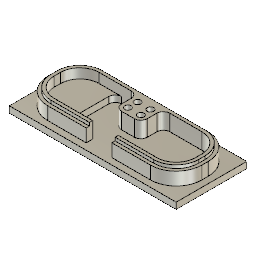
COURSERA01 (Autodesk Fusion 360 design; units mm, degrees)
Autodesk Fusion 360 part; units mm, degrees
sketch "Sketch1" plane through (0, 0, 0) normal (0, 0, 1) x (1, 0, 0)
  line L0 (-82.55, 34.925) -> (82.55, 34.925)
  line L1 (82.55, 34.925) -> (82.55, -34.925)
  line L2 (82.55, -34.925) -> (-82.55, -34.925)
  line L3 (-82.55, -34.925) -> (-82.55, 34.925)
  line L4 (-82.55, 34.925) -> (82.55, -34.925) construction
  line L5 (82.55, 34.925) -> (-82.55, -34.925) construction
  dimension "d1" = 165.1
  dimension "d2" = 69.85
  constraint horizontal L0
  constraint perpendicular L0 L1
  constraint parallel L0 L2
  constraint parallel L1 L3
  constraint coincident L4 origin
  constraint coincident L5 origin
  measures "d1" distance of L1.end L2.end
  measures "d2" distance of L0.end L1.end
extrude "Extrude1" add sketch "Sketch1" along normal blind 6.35
sketch "Sketch2" plane through (0, 0, 6.35) normal (0, 0, 1) x (-1, 0, 0)
  line L0 (82.55, 34.925) -> (-82.55, 34.925)
  line L1 (-82.55, 34.925) -> (-82.55, -34.925)
  line L2 (-82.55, -34.925) -> (82.55, -34.925)
  line L3 (82.55, -34.925) -> (82.55, 34.925)
sketch "Sketch3" plane through (0, 0, 6.35) normal (0, 0, 1) x (-1, 0, 0)
  line L0 (76.2, 28.575) -> (-76.2, 28.575)
  line L1 (-76.2, 28.575) -> (-76.2, -28.575)
  line L2 (-76.2, -28.575) -> (76.2, -28.575)
  line L3 (76.2, -28.575) -> (76.2, 28.575)
  line L4 (76.2, 28.575) -> (-76.2, -28.575) construction
  line L5 (-76.2, 28.575) -> (76.2, -28.575) construction
  dimension "d5" = 152.4
  dimension "d6" = 57.15
  constraint horizontal L0
  constraint perpendicular L0 L1
  constraint parallel L0 L2
  constraint parallel L1 L3
  constraint coincident L4 origin
  constraint coincident L5 origin
  measures "d5" distance of L1.end L2.end
  measures "d6" distance of L0.start L2.end
extrude "Extrude2" add sketch "Sketch3" along normal blind 12.7
sketch "Sketch4" plane through (0, 0, 19.05) normal (0, 0, 1) x (-1, 0, 0)
  line L0 (76.2, -28.575) -> (76.2, 28.575)
  line L1 (76.2, 28.575) -> (-76.2, 28.575)
  line L2 (-76.2, 28.575) -> (-76.2, -28.575)
  line L3 (-76.2, -28.575) -> (76.2, -28.575)
fillet "Fillet1" radius 25.4 4 edges at (-76.2, -28.575, 12.7) (76.2, -28.575, 12.7) (76.2, 28.575, 12.7) (-76.2, 28.575, 12.7)
sketch "Sketch5" plane through (0, 0, 19.05) normal (0, 0, 1) x (-1, 0, 0)
  line L0 (-73.025, 25.4) -> (73.025, 25.4)
  line L1 (73.025, 25.4) -> (73.025, -25.4)
  line L2 (73.025, -25.4) -> (-73.025, -25.4)
  line L3 (-73.025, -25.4) -> (-73.025, 25.4)
  line L4 (-73.025, 25.4) -> (73.025, -25.4) construction
  line L5 (73.025, 25.4) -> (-73.025, -25.4) construction
  line L6 (76.2, 28.575) -> (-76.2, 28.575)
  line L7 (76.2, -28.575) -> (76.2, 28.575)
  dimension "d11" = 3.175
  dimension "d12" = 3.175
  constraint horizontal L0
  constraint perpendicular L0 L1
  constraint parallel L0 L2
  constraint parallel L1 L3
  constraint coincident L4 origin
  constraint coincident L5 origin
  measures "d11" distance of L0 L6
  measures "d12" distance of L1 L7
extrude "Extrude3" add sketch "Sketch5" along normal blind 3.175
fillet "Fillet2" radius 22.225 4 edges at (73.025, -25.4, 20.6375) (-73.025, -25.4, 20.6375) (73.025, 25.4, 20.6375) (-73.025, 25.4, 20.6375)
sketch "Sketch6" plane through (0, 0, 22.225) normal (0, 0, 1) x (-1, 0, 0)
  arc A0 (50.8, -25.4) -> (73.025, -3.175) centre (50.8, -3.175) ccw
  line L0 (73.025, -3.175) -> (73.025, 3.175)
  arc A1 (73.025, 3.175) -> (50.8, 25.4) centre (50.8, 3.175) ccw
  arc A2 (-50.8, 25.4) -> (-73.025, 3.175) centre (-50.8, 3.175) ccw
  line L1 (-73.025, 3.175) -> (-73.025, -3.175)
  arc A3 (-73.025, -3.175) -> (-50.8, -25.4) centre (-50.8, -3.175) ccw
  line L2 (-50.8, -25.4) -> (50.8, -25.4)
  arc A4 (69.85, 3.175) -> (50.8, 22.225) centre (50.8, 3.175) ccw
  arc A5 (50.8, -22.225) -> (69.85, -3.175) centre (50.8, -3.175) ccw
  arc A6 (-69.85, -3.175) -> (-50.8, -22.225) centre (-50.8, -3.175) ccw
  arc A7 (-50.8, 22.225) -> (-69.85, 3.175) centre (-50.8, 3.175) ccw
  line L3 (-69.85, 3.175) -> (-69.85, -3.175)
  line L4 (69.85, 3.175) -> (69.85, -3.175)
  line L5 (50.8, -22.225) -> (12.7, -22.225)
  line L6 (50.8, 22.225) -> (12.7, 22.225)
  line L7 (-50.8, 22.225) -> (-12.7, 22.225)
  line L8 (-12.7, -22.225) -> (-50.8, -22.225)
  line L9 (12.7, -22.225) -> (12.7, 0)
  line L10 (12.7, 0) -> (-12.7, 0)
  line L11 (-12.7, 0) -> (-12.7, -22.225)
  line L12 (82.55, 34.925) -> (-82.55, 34.925)
  line L13 (12.7, 22.225) -> (12.7, 28.575)
  line L14 (-12.7, 28.575) -> (-12.7, 22.225)
  line L15 (12.7, 28.575) -> (-12.7, 28.575)
  line L16 (76.2, 28.575) -> (-76.2, 28.575)
  line L17 (34.925, -22.225) -> (34.925, 22.225)
  dimension "d17" = 19.05
  dimension "d18" = 19.05
  dimension "d19" = 19.05
  dimension "d20" = 19.05
  dimension "d21" = 19.05
  dimension "d28" = 38.1
  dimension "d29" = 38.1
  dimension "d30" = 25.4
  dimension "d31" = 34.925
  dimension "d35" = 6.35
  dimension "d36" = 44.45
  dimension "d37" = 22.225
  constraint coincident A1.centre A4.centre
  constraint coincident A0.centre A5.centre
  constraint coincident A3.centre A6.centre
  constraint coincident A2.centre A7.centre
  constraint tangent A6 L3
  constraint tangent A5 L4
  constraint tangent A5 L5
  constraint perpendicular L4 L5
  constraint vertical A4.end A5.start
  constraint vertical A6.end A7.start
  constraint tangent A4 L6
  constraint vertical L7.end L8.start
  constraint perpendicular L5 L9
  constraint perpendicular L9 L10
  constraint parallel L9 L11
  constraint vertical L5.end L6.end
  constraint parallel L7 L8
  constraint horizontal L5.end L8.start
  constraint parallel L13 L14
  constraint perpendicular L14 L15
  constraint vertical L13
  constraint coincident L5 L17.start
  constraint perpendicular L5 L17
  constraint coincident L6 L17.end
  measures "d17" distance of A0.centre A5.end
  measures "d18" distance of A1.centre A4.start
  measures "d19" horizontal distance of A2.centre A7.end
  measures "d20" distance of A3.centre A6.start
  measures "d21" radius of A7
  measures "d28" distance of A4.end L6.end
  measures "d29" horizontal distance of A7.start L7.end
  measures "d30" horizontal distance of L6.end L7.end
  measures "d31" distance of L10 L12
  measures "d35" distance of L6.end L13.end
  measures "d36" distance of L17.start L17.end
  measures "d37" distance of L9 L17
extrude "Extrude4" cut sketch "Sketch6" against normal blind 15.875 contours A6 A7 L3 L5 L6 L7 L8 L9 L10 L11 L13 L14 L15 L16 L17
extrude "Extrude5" cut sketch "Sketch6" against normal blind 9.525 contours A4 A5 L4 L5 L6 L17
fillet "Fillet3" radius 6.35 6 edges at (-34.925, 22.225, 9.525) (-34.925, -22.225, 9.525) (12.7, 0, 14.2875) (12.7, 22.225, 14.2875) (-12.7, 0, 14.2875) (-12.7, 22.225, 14.2875)
sketch "Sketch7" plane through (0, 0, 22.225) normal (0, 0, 1) x (-1, 0, 0)
  arc A0 (12.7, -6.35) -> (6.35, 0) centre (6.35, -6.35) ccw
  line L0 (6.35, 0) -> (-6.35, 0)
  arc A1 (-6.35, 0) -> (-12.7, -6.35) centre (-6.35, -6.35) ccw
  line L1 (-12.7, -6.35) -> (-12.7, -15.875)
  arc A2 (-19.05, -22.225) -> (-12.7, -15.875) centre (-19.05, -15.875) ccw
  line L2 (-19.05, -22.225) -> (-50.8, -22.225)
  arc A3 (-69.85, -3.175) -> (-50.8, -22.225) centre (-50.8, -3.175) ccw
  line L3 (-69.85, -3.175) -> (-69.85, 3.175)
  arc A4 (-50.8, 22.225) -> (-69.85, 3.175) centre (-50.8, 3.175) ccw
  line L4 (-50.8, 22.225) -> (-12.7, 22.225)
  line L5 (-12.7, 22.225) -> (-12.7, 25.4)
  line L6 (-12.7, 25.4) -> (-50.8, 25.4)
  arc A5 (-50.8, 25.4) -> (-73.025, 3.175) centre (-50.8, 3.175) ccw
  line L7 (-73.025, 3.175) -> (-73.025, -3.175)
  arc A6 (-73.025, -3.175) -> (-50.8, -25.4) centre (-50.8, -3.175) ccw
  line L8 (-50.8, -25.4) -> (50.8, -25.4)
  arc A7 (50.8, -25.4) -> (73.025, -3.175) centre (50.8, -3.175) ccw
  line L9 (73.025, -3.175) -> (73.025, 3.175)
  arc A8 (73.025, 3.175) -> (50.8, 25.4) centre (50.8, 3.175) ccw
  line L10 (50.8, 25.4) -> (12.7, 25.4)
  line L11 (12.7, 25.4) -> (12.7, 22.225)
  line L12 (12.7, 22.225) -> (50.8, 22.225)
  arc A9 (69.85, 3.175) -> (50.8, 22.225) centre (50.8, 3.175) ccw
  line L13 (69.85, 3.175) -> (69.85, -3.175)
  arc A10 (50.8, -22.225) -> (69.85, -3.175) centre (50.8, -3.175) ccw
  line L14 (50.8, -22.225) -> (19.05, -22.225)
  arc A11 (12.7, -15.875) -> (19.05, -22.225) centre (19.05, -15.875) ccw
  line L15 (12.7, -15.875) -> (12.7, -6.35)
  circle A12 centre (6.35, -15.875) radius 3.175
  circle A13 centre (-6.35, -15.875) radius 3.175
  circle A14 centre (-6.35, -6.35) radius 3.175
  circle A15 centre (6.35, -6.35) radius 3.175
  dimension "d46" = 9.525
  dimension "d53" = 6.35
  dimension "d54" = 6.35
  dimension "d55" = 6.35
  dimension "d56" = 6.35
  constraint concentric A0 A15
  constraint concentric A1 A14
  constraint vertical A12.centre A0.centre
  constraint vertical A13.centre A1.centre
  constraint horizontal A12.centre A13.centre
  measures "d46" distance of A12.centre A0.centre
  measures "d53" diameter of A12
  measures "d54" diameter of A15
  measures "d55" diameter of A13
  measures "d56" diameter of A14
extrude "Extrude6" cut sketch "Sketch7" against normal blind 22.225 contours A12 | A13 | A14 | A15
sketch "Sketch8" plane through (0, 0, 12.7) normal (0, 0, 1) x (-1, 0, 0)
  arc A0 (50.8, -22.225) -> (69.85, -3.175) centre (50.8, -3.175) ccw
  line L0 (69.85, -3.175) -> (69.85, 3.175)
  arc A1 (69.85, 3.175) -> (50.8, 22.225) centre (50.8, 3.175) ccw
  line L1 (50.8, 22.225) -> (28.575, 22.225)
  arc A2 (34.925, 15.875) -> (28.575, 22.225) centre (28.575, 15.875) ccw
  line L2 (34.925, 15.875) -> (34.925, -15.875)
  arc A3 (28.575, -22.225) -> (34.925, -15.875) centre (28.575, -15.875) ccw
  line L3 (28.575, -22.225) -> (50.8, -22.225)
